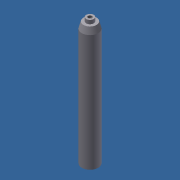
# Autodesk Inventor part: kinect standoff
Saved by Autodesk Inventor 2012 (Build 160160000, 160)
## iProperties
Created: 2012-07-17
Part Number: kinect standoff
Material: Aluminum-6061
Document SubType Name: Modeling
Designer: Ed
Density: 2.71 g/cm^3
Mass: 21.4158 g
Surface Area: 33.5258 cm^2
Volume: 7.90249 cm^3
Author: Ed
Autodesk Inventor part; units mm, degrees
ref_plane "YZ Plane" through (0, 0, 0) normal (1, 0, 0) x (0, 1, 0)
ref_plane "XZ Plane" through (0, 0, 0) normal (0, 1, 0) x (-1, 0, 0)
ref_plane "XY Plane" through (0, 0, 0) normal (0, 0, 1) x (1, 0, 0)
sketch "Sketch1" plane through (0, 0, 0) normal (0, 0, 1) x (1, 0, 0)
  line L0 (0, 0) -> (0, 85.852)
  line L1 (0, 85.852) -> (2.54, 85.852)
  line L2 (2.54, 85.852) -> (2.54, 83.312)
  line L3 (5.5626, 79.0463) -> (5.5626, 0)
  line L4 (5.5626, 0) -> (0, 0)
  line L5 (2.54, 83.312) -> (4.4196, 83.312)
  line L6 (4.4196, 83.312) -> (5.5626, 79.0463)
  dimension "d0" = 83.312
  dimension "d1" = 2.54
  dimension "d2" = 75
  dimension "d3" = 1.143
  dimension "d4" = 5.5626
  dimension "d5" = 2.54
  constraints: 14 end point, 4 parallel, 1 perpendicular, 1 vertical
  measures "d0" distance between parallel lines of L4 L5
  measures "d1" distance between parallel lines of L5 L1
  measures "d2" angle of L6 L5
  measures "d3" horizontal distance of L5.end L3.start
  measures "d4" distance between parallel lines of L0 L3
  measures "d5" distance between parallel lines of L0 L2
revolve "Revolution1" add sketch "Sketch1" angle 360 about axis through (0, 0, 0) along (0, 1, 0)
hole "Hole1" at (0, 0, 0) direction (0, 1, 0) diameter 2.6416 depth 15.0876 tip angle 118 thread size "6-32 UNC" class "2B" standard "ANSI Unified Screw Threads"
hole "Hole2" at (0, 85.852, 0) direction (0, -1, 0) diameter 2.6416 depth 15.0876 tip angle 118 thread size "6-32 UNC" class "2B" standard "ANSI Unified Screw Threads"
body "Solid1"
